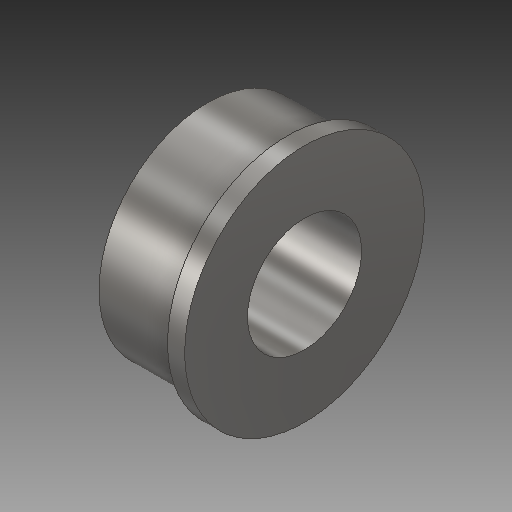
# Autodesk Inventor part: F63800
Saved by Autodesk Inventor 2019.4 (Build 234330000, 330)
## iProperties
Created: 2019-12-07
Part Number: F63800
Material: Steel, Alloy
Document SubType Name: Modeling
Designer: Mark
Mass: 14.1973 g
Surface Area: 13.1947 cm^2
Volume: 1.83665 cm^3
Density: 7.73 g/cm^3
Appearance: Semi-Polished
Author: Mark
Autodesk Inventor part; units mm, degrees
ref_plane "YZ Plane" through (0, 0, 0) normal (1, 0, 0) x (0, 1, 0)
ref_plane "XZ Plane" through (0, 0, 0) normal (0, 1, 0) x (-1, 0, 0)
ref_plane "XY Plane" through (0, 0, 0) normal (0, 0, 1) x (1, 0, 0)
sketch "Sketch1" plane through (0, 0, 0) normal (1, 0, 0) x (0, 1, 0)
  circle A0 centre (0, 0) radius 5
  circle A1 centre (0, 0) radius 9.5
  dimension "d0" = 10
  dimension "d1" = 19
  constraints: 2 centre point, 2 coincident
  measures "d0" diameter of A0
  measures "d1" diameter of A1
extrude "Extrusion1" add sketch "Sketch1" along normal blind 7
sketch "Sketch2" plane through (7, 0, 0) normal (1, 0, 0) x (0, 0, -1)
  circle A0 centre (0, 0) radius 5
  circle A1 centre (0, 0) radius 10.5
  dimension "d4" = 10
  dimension "d5" = 21
  constraints: 2 centre point, 2 coincident
  measures "d4" diameter of A0
  measures "d5" diameter of A1
extrude "Extrusion2" add sketch "Sketch2" along normal blind 1.5
body "Solid1"
